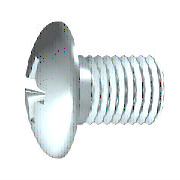
# Autodesk Inventor part: ANSI B18.6.3 - No. 1 - 64 - 3/16
Saved by Autodesk Inventor 2013 (Build 170138000, 138)
## iProperties
Created: 2010-02-08
Part Number: ANSI B18.6.3 - No. 1 - 64 - 3/16
Material: Steel, Mild
Description: Cross Recessed Pan Head Machine Screw - Type I
Document SubType Name: Modeling
Standard: ANSI B18.6.3
Designer: Phil
Standard Revision: 2003
Standards Organization: ANSI
Language: en-US
Size Designation: No. 1 - 64 - 3/16
Categories: <MemberInstance><Categories><Category DisplayName="Fasteners" InternalName="e4da775c-781d-43d5-af7c-5136215cf5a6" Mnemonic="FSTN"><Category DisplayName="Bolts" InternalName="536e6df0-f778-49ac-b2f2-25c71d2aa0b2" Mnemonic="SCRW"><CategoryParameter DisplayName="Nominal Diameter" InternalName="8bbe3f8e-44cf-40a9-a251-3a6edc8168d6" Mnemonic="nomdia"/><CategoryParameter DisplayName="Nominal Length" InternalName="238ecbaf-3e6c-45dd-aa95-4068c8e0fd02" Mnemonic="nomlen"/><CategoryParameter DisplayName="Thread Series Designation" InternalName="87c5849c-b3a5-4c3e-9c9b-2feecef9be86" Mnemonic="thrserdsgn"/><CategoryParameter DisplayName="Thread Class" InternalName="ebc0d23b-2cc6-4d2a-b376-d52aae53bab6" Mnemonic="thrclss"/><CategoryParameter DisplayName="Thread Designation" InternalName="586d5e89-370a-4089-914f-0110033585c7" Mnemonic="thrdesign"/><CategoryParameter DisplayName="Thread Type" InternalName="b4bbb7bc-d6aa-4c9f-a9a9-4152b9f6fe49" Mnemonic="thrtype"/><CategoryParameter DisplayName="Threads per Unit" InternalName="bdc6e7d2-ffd0-4d9c-a173-16b95ebb912d" Mnemonic="thrperunit1"/><CategoryParameter DisplayName="Thread Pitch" InternalName="bb82302e-82d8-4176-8fc1-c5d7bb17d5ad" Mnemonic="pitch1"/><CategoryParameter DisplayName="Nominal Diameter Designation" InternalName="03caf894-eafd-4c09-a035-916ac084b87b" Mnemonic="nomdiadesig"/><Category DisplayName="Round Head" InternalName="df3578aa-538f-4805-96a8-2439eb0c3cf7" Mnemonic="RNDSCRW"><CategoryParameter DisplayName="Shank Diameter" InternalName="c22f1a48-b8d5-43ef-ac5e-546ba91c0bd6" Mnemonic="grpdia"/><CategoryParameter DisplayName="Grip Length" InternalName="2c6ace26-543b-4217-91c4-9cdf8c3ec6f1" Mnemonic="grplen"/><CategoryParameter DisplayName="Thread Length" InternalName="a1e5edc5-4ca7-4847-8786-65b14d35af16" Mnemonic="thrlen"/><CategoryParameter DisplayName="Head Diameter" InternalName="e71ee7a1-06fd-425c-ba3b-09769885677c" Mnemonic="headdia"/><CategoryParameter DisplayName="Head Height" InternalName="2d152238-84fe-49ae-94c3-3fee884c292b" Mnemonic="headh"/><CategoryParameter DisplayName="Property Class" InternalName="85496db6-1567-48ed-b0d4-aa1f03366005" Mnemonic="propclss"/></Category></Category></Category><Category DisplayName="DataType" InternalName="23b78d0f-2648-40c6-8793-ca6db495c9e8" Mnemonic="DATATYPE"><CategoryParameter DisplayName="DisplayName" InternalName="05415f3d-3907-474b-a020-eb9d644f4cf3" Mnemonic="DISPLAYNAME"/><CategoryParameter DisplayName="InternalName" InternalName="cf1d0246-76d9-4b4a-8305-fa0409afb5c1" Mnemonic="INTERNALNAME"/><CategoryParameter DisplayName="Folder Name" InternalName="3f06958e-8713-4116-9be7-ed6184ecc97b" Mnemonic="FOLDERNAME"/><CategoryParameter DisplayName="Family Version" InternalName="914462f6-6e19-4b14-ba84-155b9680b1d0" Mnemonic="FAMILYREVISION"/><CategoryParameter DisplayName="ClipFormat" InternalName="bc51e27b-3422-4e78-93ef-cec197ddf230" Mnemonic="CLIPFORMAT"/><CategoryParameter DisplayName="IsMetric" InternalName="e2385c5b-1ea4-4823-96a8-8de651266ec3" Mnemonic="ISMETRIC"/><CategoryParameter DisplayName="Description" InternalName="13903e3d-64b1-4950-80da-f627842ea37f" Mnemonic="DESCRIPTION"/><CategoryParameter DisplayName="StdsOrg" InternalName="8f5914e1-4693-403f-8ab5-d37768198c9d" Mnemonic="STDSORG"/><CategoryParameter DisplayName="Standard" InternalName="0c0a119c-1e12-4c84-803f-101930972f5e" Mnemonic="STANDARD"/><CategoryParameter DisplayName="Manufacturer" InternalName="cd6c7a72-a28a-4e50-99a9-2c7f4e13e5ad" Mnemonic="MANUFACTURER"/><CategoryParameter DisplayName="Member Revision" InternalName="a65d44b9-392f-4f4f-857b-e4b3d54996fe" Mnemonic="MEMBERREVISION"/><CategoryParameter DisplayName="Standard Revision" InternalName="91d5a463-65c2-4fde-b823-3b7fea5e8e17" Mnemonic="STANDARDREVISION"/><CategoryParameter DisplayName="Revision Guid" InternalName="45a75005-10b1-4dfc-8d6d-dfe629f0b93c" Mnemonic="REVISIONGUID"/><CategoryParameter DisplayName="Designation" InternalName="2675968c-4ce5-49e0-a4f5-552d29089031" Mnemonic="DESIGNATION"/><CategoryParameter DisplayName="FileName" InternalName="8b46a4cc-9585-4fed-90c3-899f57e09a73" Mnemonic="FILENAME"/><CategoryParameter DisplayName="Default Row" InternalName="2af9ec52-faaa-4026-b378-f9fa4afca842" Mnemonic="DEFAULTROW"/><Category DisplayName="Part" InternalName="c0e0b642-3bcb-4cc8-9e80-f96d35c4afa4" Mnemonic="PART"><CategoryParameter DisplayName="Material" InternalName="818a152a-d3c3-49ca-80ee-df7d91421b8e" Mnemonic="MATERIAL"/><CategoryParameter DisplayName="Material Key" InternalName="5c9a8adb-dd2b-4535-b97f-0a94a95fe41f" Mnemonic="MATERIALKEY"/><CategoryParameter DisplayName="Part Number" InternalName="016b6077-bfbe-49bd-92c9-d8d59c39c941" Mnemonic="PARTNUMBER"/><CategoryParameter DisplayName="Stock Number" InternalName="4dba7c1c-e26c-444e-836c-b08b433409a8" Mnemonic="STOCKNUMBER"/></Category></Category><Category DisplayName="LegacyMap" InternalName="cd87c42b-3e48-431e-b5c0-1cbeb14dfe77" Mnemonic="LEGACYMAP"><CategoryParameter DisplayName="CatalogName" InternalName="d99d1e27-aa94-4de2-af4c-c348882a6f4f" Mnemonic="CATALOGNAME"/><CategoryParameter DisplayName="FamilyNumber" InternalName="e705e1f4-09cb-413e-91f9-551b4188271e" Mnemonic="FAMILYNUMBER"/><CategoryParameter DisplayName="MemberID" InternalName="8e5e0294-fc51-4c8f-b3d7-003dc5ed94f6" Mnemonic="MEMBERID"/><CategoryParameter DisplayName="unique CC member ID" InternalName="5193edd4-b2b0-4ab4-9d54-de900eee34e0" Mnemonic="CCCOOKIE"/><CategoryParameter DisplayName="unique DA member ID" InternalName="0918ad47-427f-4fed-ae26-24c81c58f590" Mnemonic="DACOOKIE"/><CategoryParameter DisplayName="Merge11 ID" InternalName="0ee8fb18-e2ed-4f39-96f6-1f4b5f50aa71" Mnemonic="MERGE11"/><CategoryParameter DisplayName="Split ID" InternalName="72b5c83c-be7f-45c4-ae51-9160ea6deb26" Mnemonic="SPLIT"/></Category></Categories><FamilyTemplate Id="sa0006"><FamilyTemplateParameters><FamilyTemplateParameter ObjectType="kUserParameterObject" ValueType="xs:double" Id="1" ObjectReferenceKey="KKR"/><FamilyTemplateParameter ObjectType="kUserParameterObject" ValueType="xs:double" Id="2" ObjectReferenceKey="SPD"/><FamilyTemplateParameter ObjectType="kUserParameterObject" ValueType="xs:double" Id="3" ObjectReferenceKey="KOD"/><FamilyTemplateParameter ObjectType="kUserParameterObject" ValueType="xs:double" Id="4" ObjectReferenceKey="SBR"/><FamilyTemplateParameter ObjectType="kUserParameterObject" ValueType="xs:double" Id="5" ObjectReferenceKey="KR"/><FamilyTemplateParameter ObjectType="kUserParameterObject" ValueType="xs:double" Id="6" ObjectReferenceKey="SDM"/><FamilyTemplateParameter ObjectType="kUserParameterObject" ValueType="xs:double" Id="7" ObjectReferenceKey="THREADDIA"/><FamilyTemplateParameter ObjectType="kUserParameterObject" ValueType="xs:double" Id="8" ObjectReferenceKey="GEL"/><FamilyTemplateParameter ObjectType="kUserParameterObject" ValueType="xs:double" Id="9" ObjectReferenceKey="INTI"/><FamilyTemplateParameter ObjectType="kUserParameterObject" ValueType="xs:double" Id="10" ObjectReferenceKey="BDM"/><FamilyTemplateParameter ObjectType="kUserParameterObject" ValueType="xs:double" Id="11" ObjectReferenceKey="NLG"/><FamilyTemplateParameter ObjectType="kUserParameterObject" ValueType="xs:double" Id="12" ObjectReferenceKey="KOH"/><FamilyTemplateParameter ObjectType="kUserParameterObject" ValueType="xs:double" Id="13" ObjectReferenceKey="TPU"/><FamilyTemplateParameter ObjectType="kUserParameterObject" ValueType="xs:double" Id="14" ObjectReferenceKey="PTC"/><FamilyTemplateParameter ObjectType="kUserParameterObject" ValueType="xs:double" Id="15" ObjectReferenceKey="NND"/><FamilyTemplateParameter ObjectType="kUserParameterObject" ValueType="xs:double" Id="16" ObjectReferenceKey="GUL"/><FamilyTemplateParameter ObjectType="kUserParameterObject" ValueType="xs:double" Id="17" ObjectReferenceKey="GD"/><FamilyTemplateParameter ObjectType="kUserParameterObject" ValueType="xs:double" Id="18" ObjectReferenceKey="GAL"/><FamilyTemplateParameter ObjectType="kUserParameterObject" ValueType="xs:double" Id="19" ObjectReferenceKey="TOA"/><FamilyTemplateParameter ObjectType="kUserParameterObject" ValueType="xs:double" Id="20" ObjectReferenceKey="GD1"/><FamilyTemplateParameter ObjectType="kUserParameterObject" ValueType="xs:double" Id="24" ObjectReferenceKey="R"/><FamilyTemplateParameter ObjectType="kPropertyObject" ValueType="xs:string" Id="100" ObjectReferenceKey="{32853F0F-3444-11d1-9E93-0060B03C1CA6}" SubObjectId="52"/><FamilyTemplateParameter ObjectType="kPropertyObject" ValueType="xs:string" Id="105" ObjectReferenceKey="{32853F0F-3444-11d1-9E93-0060B03C1CA6}" SubObjectId="5"/><FamilyTemplateParameter ObjectType="kPartComponentDefinitionObject" ValueType="xs:string" Id="110" SubObjectId="Material"/><FamilyTemplateParameter ObjectType="kThreadFeatureObject" ValueType="xs:structure" Id="300" ObjectReferenceKey="10020000100000003d0e0000000000008000000000000000" SubObjectId="ThreadInfo"><FamilyTemplateParameter ObjectType="" ValueType="xs:string" Id="301" SubObjectId="ThreadDesignation"/><FamilyTemplateParameter ObjectType="" ValueType="xs:string" Id="302" SubObjectId="ThreadClass"/><FamilyTemplateParameter ObjectType="" ValueType="xs:string" Id="303" SubObjectId="ThreadType"/></FamilyTemplateParameter></FamilyTemplateParameters></FamilyTemplate><CategoryParameterMap><ParamToTemplateMap><ParamToTemplate CategoryParameter="//CategoryParameter[@InternalName='05415f3d-3907-474b-a020-eb9d644f4cf3']" ConstantValue="Cross Recessed Pan Head Machine Screw - Type I - Inch"/><ParamToTemplate CategoryParameter="//CategoryParameter[@InternalName='cf1d0246-76d9-4b4a-8305-fa0409afb5c1']" ConstantValue="5fc90f9e-0f01-4955-befe-e4aa7dfb21e5"/><ParamToTemplate CategoryParameter="//CategoryParameter[@InternalName='3f06958e-8713-4116-9be7-ed6184ecc97b']" ConstantValue="ANSI B18.6.3(24)"/><ParamToTemplate CategoryParameter="//CategoryParameter[@InternalName='914462f6-6e19-4b14-ba84-155b9680b1d0']" ConstantValue="10"/><ParamToTemplate CategoryParameter="//CategoryParameter[@InternalName='bc51e27b-3422-4e78-93ef-cec197ddf230']" ConstantValue="CF_INVENTOR.STDPARTS"/><ParamToTemplate CategoryParameter="//CategoryParameter[@InternalName='e2385c5b-1ea4-4823-96a8-8de651266ec3']" ConstantValue="false"/><ParamToTemplate CategoryParameter="//CategoryParameter[@InternalName='13903e3d-64b1-4950-80da-f627842ea37f']" ConstantValue="Cross Recessed Pan Head Machine Screw - Type I"/><ParamToTemplate CategoryParameter="//CategoryParameter[@InternalName='8f5914e1-4693-403f-8ab5-d37768198c9d']" ConstantValue="ANSI"/><ParamToTemplate CategoryParameter="//CategoryParameter[@InternalName='0c0a119c-1e12-4c84-803f-101930972f5e']" ConstantValue="ANSI B18.6.3"/><ParamToTemplate CategoryParameter="//CategoryParameter[@InternalName='cd6c7a72-a28a-4e50-99a9-2c7f4e13e5ad']" TemplateParameter="104"/><ParamToTemplate CategoryParameter="//CategoryParameter[@InternalName='91d5a463-65c2-4fde-b823-3b7fea5e8e17']" ConstantValue="2003"/><ParamToTemplate CategoryParameter="//CategoryParameter[@InternalName='45a75005-10b1-4dfc-8d6d-dfe629f0b93c']" ConstantValue="c3d97335-2f23-4fde-a800-918efb1d6722"/><ParamToTemplate CategoryParameter="//CategoryParameter[@InternalName='2af9ec52-faaa-4026-b378-f9fa4afca842']" ConstantValue="10"/><ParamToTemplate CategoryParameter="//CategoryParameter[@InternalName='d99d1e27-aa94-4de2-af4c-c348882a6f4f']" ConstantValue="ANSI"/><ParamToTemplate CategoryParameter="//CategoryParameter[@InternalName='8b46a4cc-9585-4fed-90c3-899f57e09a73']" ConstantValue="ANSI B18.6.3 - 1-64 UNC - 0.1875(4A)"/><ParamToTemplate CategoryParameter="//CategoryParameter[@InternalName='a65d44b9-392f-4f4f-857b-e4b3d54996fe']" ConstantValue="6744ddfb-da3f-41b7-a87e-dab810c2eef7"/><ParamToTemplate CategoryParameter="//CategoryParameter[@InternalName='2c6ace26-543b-4217-91c4-9cdf8c3ec6f1']" ConstantValue="0.039062598"/><ParamToTemplate CategoryParameter="//CategoryParameter[@InternalName='ebc0d23b-2cc6-4d2a-b376-d52aae53bab6']" ConstantValue="2A"/><ParamToTemplate CategoryParameter="//CategoryParameter[@InternalName='87c5849c-b3a5-4c3e-9c9b-2feecef9be86']" ConstantValue="UNC"/><ParamToTemplate CategoryParameter="//CategoryParameter[@InternalName='03caf894-eafd-4c09-a035-916ac084b87b']" ConstantValue="#1"/><ParamToTemplate CategoryParameter="//CategoryParameter[@InternalName='b4bbb7bc-d6aa-4c9f-a9a9-4152b9f6fe49']" ConstantValue="ANSI Unified Screw Threads"/><ParamToTemplate CategoryParameter="//CategoryParameter[@InternalName='e705e1f4-09cb-413e-91f9-551b4188271e']" ConstantValue="117"/><ParamToTemplate CategoryParameter="//CategoryParameter[@InternalName='8e5e0294-fc51-4c8f-b3d7-003dc5ed94f6']" ConstantValue="10"/><ParamToTemplate CategoryParameter="//CategoryParameter[@InternalName='c22f1a48-b8d5-43ef-ac5e-546ba91c0bd6']" TemplateParameter="10"/><ParamToTemplate CategoryParameter="//CategoryParameter[@InternalName='2675968c-4ce5-49e0-a4f5-552d29089031']" TemplateParameter="100"/><ParamToTemplate CategoryParameter="//CategoryParameter[@InternalName='a1e5edc5-4ca7-4847-8786-65b14d35af16']" TemplateParameter="8"/><ParamToTemplate CategoryParameter="//CategoryParameter[@InternalName='e71ee7a1-06fd-425c-ba3b-09769885677c']" TemplateParameter="3"/><ParamToTemplate CategoryParameter="//CategoryParameter[@InternalName='2d152238-84fe-49ae-94c3-3fee884c292b']" TemplateParameter="12"/><ParamToTemplate CategoryParameter="//CategoryParameter[@InternalName='818a152a-d3c3-49ca-80ee-df7d91421b8e']" TemplateParameter="110"/><ParamToTemplate CategoryParameter="//CategoryParameter[@InternalName='238ecbaf-3e6c-45dd-aa95-4068c8e0fd02']" TemplateParameter="11"/><ParamToTemplate CategoryParameter="//CategoryParameter[@InternalName='8bbe3f8e-44cf-40a9-a251-3a6edc8168d6']" TemplateParameter="15"/><ParamToTemplate CategoryParameter="//CategoryParameter[@InternalName='016b6077-bfbe-49bd-92c9-d8d59c39c941']" TemplateParameter="105"/><ParamToTemplate CategoryParameter="//CategoryParameter[@InternalName='bb82302e-82d8-4176-8fc1-c5d7bb17d5ad']" TemplateParameter="14"/><ParamToTemplate CategoryParameter="//CategoryParameter[@InternalName='586d5e89-370a-4089-914f-0110033585c7']" TemplateParameter="301"/><ParamToTemplate CategoryParameter="//CategoryParameter[@InternalName='bdc6e7d2-ffd0-4d9c-a173-16b95ebb912d']" TemplateParameter="13"/></ParamToTemplateMap></CategoryParameterMap></MemberInstance>
Density: 7.86 g/cm^3
Mass: 0.174597 g
Surface Area: 0.586701 cm^2
Volume: 0.0222134 cm^3
IsCustomPart: 0
Author: Phil
Autodesk Inventor part; units mm, degrees
ref_plane "YZ Plane" through (0, 0, 0) normal (1, 0, 0) x (0, 1, 0)
ref_plane "XZ Plane" through (0, 0, 0) normal (0, 1, 0) x (-1, 0, 0)
sketch "Sketch1" plane through (0, 0, 0) normal (0, 0, 1) x (1, 0, 0)
  line L0 (-2.6081, 0) -> (5.9909, 0) projected
  line L1 (0, -0.3703) -> (0, 2.2217) projected
  line L2 (4.7625, 0) -> (4.7625, 0.9271)
  line L3 (4.7625, 0.9271) -> (0.9922, 0.9271)
  line L4 (-1.3462, 1.8034) -> (-1.3462, 0) construction
  arc A0 (-0.4998, 1.8034) -> (-1.2113, 0.7837) centre (0.9982, 0) ccw
  line L5 (-1.2113, 0.7837) -> (-0.7521, 0.5547)
  line L6 (-0.7521, 0.5547) -> (-0.4572, 0)
  line L7 (-0.4572, 0) -> (4.7625, 0)
  line L8 (-1.2113, 0.7837) -> (-1.3462, 0.8509) construction
  line L9 (-0.4998, 1.8034) -> (-1.3462, 1.8034)
  line L10 (-1.3462, 0) -> (-1.3462, 1.8034)
  arc A1 (-1.2113, 0.7837) -> (-1.3462, 0) centre (0.9982, 0) ccw
  line L11 (-0.4998, 1.8034) -> (0, 1.8034)
  line L12 (0, 0.9271) -> (0.5953, 0.9271)
  line L13 (0.5953, 0.9271) -> (0.9922, 0.9271)
  line L14 (0, 0.9271) -> (0, 1.8034)
  line L15 (0.9922, 0.9271) -> (0, 0.9271) construction
  dimension "d1" = 1.8542
  dimension "d2" = 0.889
  dimension "d12" = 62
  dimension "d13" = 26.5
  dimension "d16" = 1.7018
  dimension "d21" = 1.8542
  dimension "d22" = 3.7703
  dimension "d23" = 0.3969
  dimension "d24" = 1.3462
  dimension "d25" = 2.3444
  dimension "d29" = 3.6068
  dimension "d30" = 4.7625
  constraints: 28 end point, 5 collinear, 4 perpendicular, 4 point on circle, 3 parallel, 3 point on line, 2 centre point, 1 coincident, 1 tangent
  measures "d1" diameter of L3 L7
  measures "d2" distance from line of L6.end L4
  measures "d12" angle of L6 L7
  measures "d13" angle of L5 L7
  measures "d16" diameter of L8.end L7
  measures "d21" diameter of L12 L7
  measures "d22" distance of L2.end L3.end
  measures "d23" distance of L12.end L3.end
  measures "d24" distance between parallel lines of L4 L14
  measures "d25" radius of A0
  measures "d29" diameter of L9 L7
  measures "d30" distance between parallel lines of L2 L14
revolve "Body" add sketch "Sketch1" angle 360 about axis through (-0.4572, 0, 0) along (1, 0, 0) contours L6 L5 A0 L11 L1 L0 | L1 L12 L13 L3 L2 L0
ref_plane "Workplane" through (-1.3462, 0, 0) normal (1, 0, 0) x (0, 1, 0)
sketch "Sketch2" plane through (-1.3462, 0, 0) normal (1, 0, 0) x (0, 1, 0)
  circle A0 centre (0, 0) radius 1.8034 projected
  line L0 (-3.3485, 0) -> (7.4674, 0) projected
  line L1 (0, -3.3485) -> (0, 7.4674) projected
  line L2 (0, 0.8509) -> (0, 0) construction
  line L3 (0, 0) -> (0.8509, 0) construction
  line L4 (0, 0) -> (5.9223, 5.9223) construction
  arc A1 (0.2836, 0) -> (0, 0.2836) centre (0, 0) ccw construction
  arc A2 (0.8509, 0) -> (0.8321, 0.1778) centre (0, 0) ccw
  arc A3 (0.1778, 0.8321) -> (0, 0.8509) centre (0, 0) ccw
  arc A4 (0.8321, 0.1778) -> (0.1778, 0.8321) centre (0, 0) ccw
  arc A5 (0.8321, -0.1778) -> (0.8509, 0) centre (0, 0) ccw
  arc A6 (0, -0.8509) -> (0.1778, -0.8321) centre (0, 0) ccw
  arc A7 (0.1778, -0.8321) -> (0.8321, -0.1778) centre (0, 0) ccw
  arc A8 (-0.8321, 0.1778) -> (-0.8509, 0) centre (0, 0) ccw
  arc A9 (0, 0.8509) -> (-0.1778, 0.8321) centre (0, 0) ccw
  arc A10 (-0.1778, 0.8321) -> (-0.8321, 0.1778) centre (0, 0) ccw
  arc A11 (-0.1778, -0.8321) -> (0, -0.8509) centre (0, 0) ccw
  arc A12 (-0.8321, -0.1778) -> (-0.1778, -0.8321) centre (0, 0) ccw
  arc A13 (-0.8509, 0) -> (-0.8321, -0.1778) centre (0, 0) ccw
  arc A14 (0.4216, 0.0573) -> (0, 0.4254) centre (0, 0) ccw construction
  line L5 (0.8321, 0.1778) -> (0.4054, 0.1291)
  line L6 (0.1778, 0.8321) -> (0.1291, 0.4054)
  line L7 (0.1539, 0.2383) -> (0.1539, 0.2364)
  arc A15 (0.1291, 0.4054) -> (0.4054, 0.1291) centre (0.3771, 0.3771) ccw
  arc A16 (0.8321, -0.1778) -> (0.8509, 0) centre (0, 0) ccw
  arc A17 (0, -0.8509) -> (0.1778, -0.8321) centre (0, 0) ccw
  arc A18 (0.1778, -0.8321) -> (0.8321, -0.1778) centre (0, 0) ccw
  line L8 (0.8321, -0.1778) -> (0.4054, -0.1291)
  line L9 (0.1778, -0.8321) -> (0.1291, -0.4054)
  arc A19 (0.4054, -0.1291) -> (0.1291, -0.4054) centre (0.3771, -0.3771) ccw
  arc A20 (-0.8321, 0.1778) -> (-0.8509, 0) centre (0, 0) ccw
  arc A21 (0, 0.8509) -> (-0.1778, 0.8321) centre (0, 0) ccw
  arc A22 (-0.1778, 0.8321) -> (-0.8321, 0.1778) centre (0, 0) ccw
  arc A23 (-0.1778, -0.8321) -> (0, -0.8509) centre (0, 0) ccw
  arc A24 (-0.8321, -0.1778) -> (-0.1778, -0.8321) centre (0, 0) ccw
  arc A25 (-0.8509, 0) -> (-0.8321, -0.1778) centre (0, 0) ccw
  line L10 (-0.8321, 0.1778) -> (-0.4054, 0.1291)
  line L11 (-0.1778, 0.8321) -> (-0.1291, 0.4054)
  arc A26 (-0.4054, 0.1291) -> (-0.1291, 0.4054) centre (-0.3771, 0.3771) ccw
  line L12 (-0.1778, -0.8321) -> (-0.1291, -0.4054)
  arc A27 (-0.1291, -0.4054) -> (-0.4054, -0.1291) centre (-0.3771, -0.3771) ccw
  line L13 (-0.8321, -0.1778) -> (-0.4054, -0.1291)
  dimension "d4" = 45
  dimension "d5" = 0.5673
  dimension "d6" = 1.7018
  dimension "d7" = 0.1778
  dimension "d17" = 0.8509
  constraints: 57 point on circle, 27 centre point, 24 end point, 18 symmetric about line, 4 coincident, 3 collinear, 3 tangent, 2 point on line, 1 midpoint, 1 perpendicular, 27 other
  measures "d4" angle of L4 L3
  measures "d5" diameter of A1
  measures "d6" diameter of A4
  measures "d7" distance from line of L6.start L2
  measures "d17" diameter of A14
extrude "Slot" add sketch "Sketch2" along normal up to next draft 5 contours L5 A15 L6 A4 | A7 L9 A19 L8 | L11 A26 L10 A10 | A12 L13 A27 L12
revolve "Cut" cut sketch "Sketch1" angle 360 about axis through (-0.4572, 0, 0) along (1, 0, 0) contours L10 L9 A0 A1
fillet "Fillet1" radius 0.0711 5 edges at (-1.2113, 0, 0.7837) (-1.2113, 0.7796, -0.0797) (-1.2113, 0.7796, 0.0797) (-1.2113, 0, -0.7837) (-1.2113, -0.7837, 0)
thread "Thread" size "1-64 UNC" class "2A" standard "ANSI Unified Screw Threads" length 3.7703
fillet "Fillet2" radius 0.127 1 edges at (-0.4998, -1.8034, 0)
fillet "Fillet3" radius 0.0025 1 edges at (0, -0.9271, 0)
equation "\"d1\" = GD"
equation "\"d2\" = INTI"
equation "\"d16\" = SDM"
equation "\"d21\" = BDM"
equation "\"d22\" = GEL"
equation "\"d23\" = GAL"
equation "\"d24\" = KOH"
equation "\"d25\" = KR"
equation "\"d29\" = KOD"
equation "\"d30\" = NLG"
equation "\"d5\" = 0.333333 * SDM"
equation "\"d6\" = SDM"
equation "\"d7\" = 0.5 * SBR"
equation "\"d17\" = 0.5 * SDM"
equation "\"d19\" = 0.2 * SBR"
equation "\"d8\" = GEL"
equation "\"d27\" = KKR"
equation "\"d74\" = R"
equation "\"GD\" = NND"
equation "\"NLG\" = 4.7625"
equation "\"GEL\" = 3.77031"
equation "\"KOD\" = 3.6068"
equation "\"KOH\" = 1.3462"
equation "\"SDM\" = 1.7018"
equation "\"INTI\" = 0.889"
equation "\"SBR\" = 0.3556"
equation "\"d3\" = -KOH"
equation "\"GAL\" = 0.39687"
equation "\"BDM\" = NND"
equation "\"KR\" = 0.65 * KOD"
equation "\"KKR\" = 0.127"
equation "\"R\" = 0.00254"
equation "\"SPD\" = -1.35 * PTC + 0.9 * NND"
equation "\"THREADDIA\" = 1.8542"
equation "\"NND\" = 1.8542"
equation "\"GUL\" = 0"
equation "\"TOA\" = 30deg"
equation "\"GD1\" = 1.36727"
equation "\"PTC\" = 0.396875"
body "Solid1"
